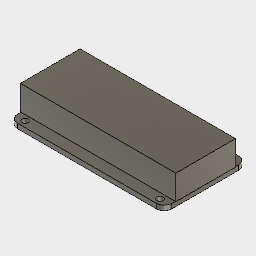
878 7-segment display backpack (Autodesk Fusion 360 design; units mm, degrees)
Autodesk Fusion 360 part; units mm, degrees
sketch "Sketch1" plane through (0, 0, 0) normal (0, 0, 1) x (1, 0, 0)
  line L0 (25.02, -13.335) -> (-25.02, -13.335)
  line L1 (-25.02, -13.335) -> (-25.02, 13.335)
  line L2 (-25.02, 13.335) -> (25.02, 13.335)
  line L3 (25.02, 13.335) -> (25.02, -13.335)
  line L4 (25.02, -13.335) -> (-25.02, 13.335) construction
  line L5 (-25.02, -13.335) -> (25.02, 13.335) construction
  circle A0 centre (-21.844, 11.43) radius 1
  circle A1 centre (21.846, 11.43) radius 1
  line L6 (0, 0) -> (25.02, 0) construction
  circle A2 centre (-21.844, -11.43) radius 1
  circle A3 centre (21.846, -11.43) radius 1
  dimension "d1" = 26.67
  dimension "d2" = 50.04
  dimension "d3" = 2
  dimension "d4" = 11.43
  dimension "d5" = 21.844
  dimension "d7" = 43.69
  measures "d1" distance of L0.end L1.end
  measures "d2" distance of L1.end L2.end
  measures "d3" diameter of A0
  measures "d4" distance of L6.start A0.centre
  measures "d5" distance of L6.start A0.centre
  measures "d7" distance of A0.centre A1.centre
extrude "Extrude1" add sketch "Sketch1" along normal blind 1.6 makes body 1
fillet "Fillet1" radius 2.54 4 edges at (-25.02, 13.335, 0.8) (-25.02, -13.335, 0.8) (25.02, 13.335, 0.8) (25.02, -13.335, 0.8) on bodies 1
sketch "Sketch2" plane through (0, 0, 1.6) normal (0, 0, 1) x (-1, 0, 0)
  arc A0 (-22.48, 13.335) -> (-25.02, 10.795) centre (-22.48, 10.795) ccw
  line L0 (-25.02, 10.795) -> (-25.02, -10.795) construction
  arc A1 (-25.02, -10.795) -> (-22.48, -13.335) centre (-22.48, -10.795) ccw
  line L1 (-22.48, -13.335) -> (22.48, -13.335)
  arc A2 (22.48, -13.335) -> (25.02, -10.795) centre (22.48, -10.795) ccw
  line L2 (25.02, -10.795) -> (25.02, 10.795) construction
  arc A3 (25.02, 10.795) -> (22.48, 13.335) centre (22.48, 10.795) ccw
  line L3 (22.48, 13.335) -> (-22.48, 13.335)
  circle A4 centre (-21.846, 11.43) radius 1 construction
  circle A5 centre (21.844, 11.43) radius 1 construction
  circle A6 centre (-21.846, -11.43) radius 1 construction
  circle A7 centre (21.844, -11.43) radius 1 construction
  line L4 (-25.2, 9.7) -> (25.2, 9.7)
  line L5 (25.2, 9.7) -> (25.2, -9.7)
  line L6 (25.2, -9.7) -> (-25.2, -9.7)
  line L7 (-25.2, -9.7) -> (-25.2, 9.7)
  line L8 (-25.2, 9.7) -> (25.2, -9.7) construction
  line L9 (25.2, 9.7) -> (-25.2, -9.7) construction
  line L10 (-25.5, 10) -> (25.5, 10)
  line L11 (25.5, 10) -> (25.5, -10)
  line L12 (25.5, -10) -> (-25.5, -10)
  line L13 (-25.5, -10) -> (-25.5, 10)
  dimension "d11" = 50.4
  dimension "d12" = 19.4
  dimension "d28" = 0.3
  measures "d11" distance of L5.end L6.end
  measures "d12" distance of L4.end L5.end
extrude "Extrude2" add sketch "Sketch2" along normal blind 8 separate body contours L4 L5 L6 L7 makes body 2
sketch "Sketch3" plane through (0, 0, 1.6) normal (0, 0, 1) x (-1, 0, 0)
  arc A0 (-22.48, 13.335) -> (-25.02, 10.795) centre (-22.48, 10.795) ccw
  line L0 (-25.02, 10.795) -> (-25.02, -10.795)
  arc A1 (-25.02, -10.795) -> (-22.48, -13.335) centre (-22.48, -10.795) ccw
  line L1 (-22.48, -13.335) -> (22.48, -13.335)
  arc A2 (22.48, -13.335) -> (25.02, -10.795) centre (22.48, -10.795) ccw
  line L2 (25.02, -10.795) -> (25.02, 10.795)
  arc A3 (25.02, 10.795) -> (22.48, 13.335) centre (22.48, 10.795) ccw
  line L3 (22.48, 13.335) -> (-22.48, 13.335)
  circle A4 centre (-21.846, 11.43) radius 1
  circle A5 centre (21.844, 11.43) radius 1
  circle A6 centre (-21.846, -11.43) radius 1
  circle A7 centre (21.844, -11.43) radius 1
  circle A8 centre (21.844, -11.43) radius 1.9
  circle A9 centre (-21.846, -11.43) radius 1.9
  circle A10 centre (21.844, 11.43) radius 1.9
  circle A11 centre (-21.846, 11.43) radius 1.9
  line L4 (27.52, -10.795) -> (27.52, 10.795)
  arc A12 (27.52, 10.795) -> (22.48, 15.835) centre (22.48, 10.795) ccw
  line L5 (22.48, 15.835) -> (-22.48, 15.835)
  arc A13 (-22.48, 15.835) -> (-27.52, 10.795) centre (-22.48, 10.795) ccw
  line L6 (-27.52, 10.795) -> (-27.52, -10.795)
  arc A14 (-27.52, -10.795) -> (-22.48, -15.835) centre (-22.48, -10.795) ccw
  line L7 (-22.48, -15.835) -> (22.48, -15.835)
  arc A15 (22.48, -15.835) -> (27.52, -10.795) centre (22.48, -10.795) ccw
  dimension "d15" = 3.8
  dimension "d16" = 3.8
  dimension "d17" = 3.8
  dimension "d18" = 3.8
  dimension "d19" = 2.5
  measures "d15" diameter of A8
  measures "d16" diameter of A9
  measures "d17" diameter of A10
  measures "d18" diameter of A11
extrude "Extrude3" add sketch "Sketch3" along normal blind 4 and the other way blind -3 separate body contours A0 L0 A1 L1 A2 L2 A3 L3 | A4 | A5 | A6 | A7 | A8 | A9 | A10 | A11 | L4 A12 L5 A13 L6 A14 L7 A15 makes body 3
extrude "Extrude4" add sketch "Sketch3" along normal blind 3 contours A4 | A5 | A6 | A7 | A8 | A9 | A10 | A11 bodies 3
extrude "Extrude5" add sketch "Sketch3" against normal blind 2 contours A4 | A5 | A6 | A7 bodies 3
extrude "Extrude6" cut sketch "Sketch2" along normal through all contours L4 L5 L6 L7 | L10 L11 L12 L13 bodies 3
hidden bodies 3
